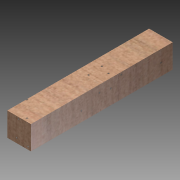
# Autodesk Inventor part: Front Spacer
Saved by Autodesk Inventor 2012 (Build 160160000, 160)
## iProperties
Created: 2013-03-14
Part Number: Front Spacer
Material: Wood (Cherry)
Document SubType Name: Modeling
Designer: fixer
Mass: 6.14515 g
Surface Area: 41.9354 cm^2
Volume: 12.2903 cm^3
Density: 0.5 g/cm^3
Author: fixer
Autodesk Inventor part; units mm, degrees
ref_plane "YZ Plane" through (0, 0, 0) normal (1, 0, 0) x (0, 1, 0)
ref_plane "XZ Plane" through (0, 0, 0) normal (0, 1, 0) x (-1, 0, 0)
ref_plane "XY Plane" through (0, 0, 0) normal (0, 0, 1) x (1, 0, 0)
sketch "Sketch1" plane through (0, 0, 0) normal (0, 0, 1) x (1, 0, 0)
  line L0 (-6.35, -6.35) -> (6.35, -6.35)
  line L1 (6.35, -6.35) -> (6.35, 6.35)
  line L2 (6.35, 6.35) -> (-6.35, 6.35)
  line L3 (-6.35, 6.35) -> (-6.35, -6.35)
  point P0 (0, 0)
  point P1 (6.35, 0)
  point P2 (0, -6.35)
  dimension "d0" = 12.7
  dimension "d1" = 12.7
  constraints: 8 end point, 2 midpoint, 2 parallel, 1 horizontal, 1 horizontal alignment, 1 perpendicular, 1 vertical alignment
  measures "d0" distance of L1.end L2.end
  measures "d1" distance of L2.end L0.start
extrude "Extrusion1" add sketch "Sketch1" along normal mid plane 76.2
body "Solid1"
